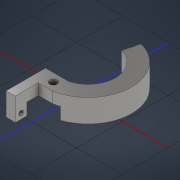
# Autodesk Inventor part: holder2_base
Saved by Autodesk Inventor 2021 (Build 250183000, 183)
## iProperties
Created: 2021-06-04
Part Number: holder2_base
Material: Steel, Mild
Document SubType Name: Modeling
Designer: Watchdog
Density: 7.85 g/cm^3
Appearance: Semi-Polished
Author: Watchdog
Autodesk Inventor part; units mm, degrees
ref_plane "YZ Plane" through (0, 0, 0) normal (1, 0, 0) x (0, 1, 0)
ref_plane "XZ Plane" through (0, 0, 0) normal (0, 1, 0) x (-1, 0, 0)
sketch "clawBase" plane through (0, 0, 0) normal (0, 1, 0) x (-1, 0, 0)
  line L0 (-3, -16.619) -> (0, -5)
  line L1 (0, -5) -> (0, 7)
  arc A0 (0, 7) -> (-3, -16.619) centre (0, -5) ccw
  arc A1 (0, 14) -> (-4.75, -23.3967) centre (0, -5) ccw
  line L2 (-3, -16.619) -> (-4.75, -23.3967)
  line L3 (0, 7) -> (0, 14)
  line L4 (0, 0) -> (0, 12)
  dimension "d3" = 12
  dimension "d5" = 7
  dimension "d6" = 0
  dimension "d7" = 5
  dimension "d8" = 3
  dimension "d11" = 12
  dimension "d12" = 0
  constraints: 10 end point, 6 point on circle, 2 centre point, 2 collinear, 1 coincident, 1 vertical
  measures "d3" distance of L0.start L0.end
  measures "d5" radial gap between concentric circles of A1 A0
  measures "d6" horizontal distance of L0.end L4.start
  measures "d7" distance of L4.start L0.end
  measures "d8" horizontal distance of L4.start L0.start
  measures "d11" distance of L4.start L4.end
  measures "d12" distance between parallel lines of L4 L1
extrude "clamp" add sketch "clawBase" against normal blind 10 contours L2 A1 L3 A0
ref_plane "reduction" through (3, 0, 7) normal (-1, 0, 0) x (0, 0, 1)
split "reductionSplit" plane through (3, 0, 7) removes the side toward (-1, 0, 0)
sketch "Sketch7" plane through (3, -10, 6.619) normal (-1, 0, 0) x (0, 0, 1)
  line L0 (0, 0) -> (0, 10) projected
  line L1 (7.1427, 0) -> (0, 0) projected
  line L2 (7.1427, 10) -> (7.1427, 0) projected
  line L3 (0, 10) -> (7.1427, 10) projected
  point P0 (-6.619, 10)
extrude "arm_c" add sketch "Sketch7" along normal blind 10
sketch "Sketch8" plane through (-7, 0, 13.7617) normal (0, 0, 1) x (1, 0, 0)
  line L0 (10, -10) -> (0, -10) projected
  line L1 (0, 0) -> (4, 0)
  line L2 (4, 0) -> (4, -10)
  line L3 (4, -10) -> (0, -10)
  line L4 (0, -10) -> (0, 0)
  point P0 (7, 0)
  dimension "d35" = 4
  constraints: 8 end point, 2 parallel, 1 horizontal, 1 perpendicular, 1 point on line
  measures "d35" distance between parallel lines of L4 L2
extrude "arb_b" add sketch "Sketch8" along normal blind 10
sketch "Sketch9" plane through (0, 0, 0) normal (0, 1, 0) x (1, 0, 0)
  line L0 (3, -6.619) -> (-7, -6.619) projected
  line L1 (3, -13.7617) -> (-3, -13.7617) projected
  point P0 (0, 0)
  point P1 (0, -10.1903)
  dimension "d39" = 7.1427
  dimension "d41" = 0
  dimension "d42" = 3.5714
  measures "d39" distance between parallel lines of L0 L1
  measures "d41" horizontal distance of point (0, 0) point (0, -10.19)
  measures "d42" distance from line of L0 point (0, -10.19)
hole "pinHole" at (0, 0, 10.1903) direction (0, -1, 0) diameter 3.25 end through all
sketch "Sketch10" plane through (3, -10, 6.619) normal (0, 0, -1) x (-1, 0, 0)
  line L0 (10, 10) -> (10, 0) projected
  line L1 (-3, 0) -> (10, 0)
  line L2 (10, 0) -> (10, 5.25)
  line L3 (10, 5.25) -> (-3, 5.25)
  line L4 (-3, 5.25) -> (-3, 0)
  line L5 (0, 10) -> (0, 0) projected
  line L6 (0, 0) -> (6, 0) projected
  point P0 (3, 10)
  point P1 (10, 0)
  dimension "d50" = 5.25
  dimension "d64" = 3
  dimension "d65" = 0
  constraints: 8 end point, 2 parallel, 1 horizontal, 1 perpendicular, 1 point on line
  measures "d50" distance between parallel lines of L1 L3
  measures "d64" distance between parallel lines of L5 L4
  measures "d65" distance between parallel lines of L6 L1
extrude "halfcut" cut sketch "Sketch10" along normal blind 4.25 and the other way blind 19.75
sketch "Sketch12" plane through (-7, -4.75, 6.619) normal (0, -1, 0) x (1, 0, 0)
  line L0 (0, 0) -> (0, 17.1427) projected
  line L1 (4, 7.1427) -> (4, 17.1427) projected
  line L2 (0, 17.1427) -> (4, 17.1427)
  line L3 (4, 17.1427) -> (4, 12.1427)
  line L4 (4, 12.1427) -> (0, 12.1427)
  line L5 (0, 12.1427) -> (0, 17.1427)
  line L6 (4, 7.1427) -> (10, 7.1427) projected
  point P0 (7, -6.619)
  point P1 (0, 12.1427)
  dimension "d68" = 5
  constraints: 8 end point, 2 parallel, 1 horizontal, 1 midpoint, 1 perpendicular
  measures "d68" distance between parallel lines of L4 L6
extrude "Extrusion6" add sketch "Sketch12" along normal up to surface (5.25 mm away)
sketch "Sketch11" plane through (-3, 0, 23.7617) normal (1, 0, 0) x (0, 0, -1)
  line L0 (0, -10) -> (0, 0) projected
  line L1 (5, -10) -> (0, -10) projected
  point P0 (23.7617, 0)
  point P1 (2.5, -7.625)
  dimension "d71" = 2.5
  dimension "d72" = 2.375
  measures "d71" distance from line of L0 point (2.5, -7.625)
  measures "d72" distance from line of L1 point (2.5, -7.625)
hole "cableHole" at (-3, -7.625, 21.2617) direction (-1, 0, 0) diameter 2 end through all
equation "\"d3\" = r"
equation "\"d5\" = t"
equation "\"d8\" = 0.5 * a1"
equation "\"d11\" = r"
equation "\"d42\" = 0.5 * d39"
equation "\"d43\" = dpin"
equation "\"d57\" = dcable"
equation "\"r\" = 12"
equation "\"t\" = 7"
equation "\"a1\" = 6"
equation "\"fillet\" = 0.5"
equation "\"d14\" = -0.5 * a2"
equation "\"dpin\" = 3.25"
equation "\"tpinhole\" = t - dpin"
equation "\"linkb\" = d36 + 0.5 * t - d56"
equation "\"dcable\" = 2"
equation "\"a2\" = 6"
equation "\"d36\" = 10"
equation "\"d56\" = 2.137935"
body "Solid1"
